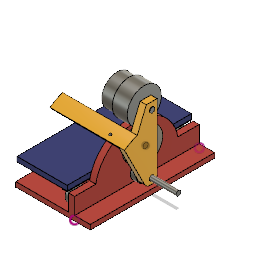
Second Design (Autodesk Fusion 360 design; units mm, degrees)
Autodesk Fusion 360 part; units mm, degrees
note: some values were not read from the file. Set by a fixed rule: which face or edge a step refers to.
sketch "Sketch1" plane through (0, 0, 0) normal (1, 0, 0) x (0, 0, -1)
  circle A0 centre (0, 0) radius 12.5
  line L0 (0, 0) -> (138.4704, 0)
  circle A1 centre (25, 0) radius 12.5
  circle A2 centre (65, 0) radius 27.5
  dimension "d1" = 25
  dimension "d2" = 25
  dimension "d3" = 55
  constraint coincident A0.centre L0.start
  constraint horizontal L0
  measures "d1" diameter of A0
  measures "d2" diameter of A1
  measures "d3" diameter of A2
extrude "Extrude1" add sketch "Sketch1" against normal blind 10 contours A0 | L0 A1 | L0 A1 makes body 1
sketch "Sketch2" plane through (0, 0, 0) normal (1, 0, 0) x (0, 0, -1)
  circle A0 centre (25, 0) radius 12.5
  line L0 (0, 0) -> (94.7994, 0)
  circle A1 centre (65, 0) radius 27.5
  dimension "d6" = 55
  constraint coincident L0.start origin
  constraint horizontal L0
  measures "d6" diameter of A1
extrude "Extrude2" add sketch "Sketch2" against normal blind 24 separate body contours L0 A1 | L0 A1 makes body 2
sketch "Sketch3" plane through (-24, 0, 0) normal (-1, 0, 0) x (0, 0, 1)
  circle A0 centre (-65, 0) radius 27.5
  circle A1 centre (-65, 0) radius 24.6188
  constraint concentric A0 A1
extrude "Extrude3" add sketch "Sketch3" along normal blind 20 contours A1 bodies 2
sketch "Sketch4" plane through (-10, 0, 0) normal (-1, 0, 0) x (0, 0, 1)
  circle A0 centre (0, 0) radius 12.5
  circle A1 centre (0, 0) radius 4
  dimension "d11" = 8
  constraint coincident A0.centre A1.centre
  measures "d11" diameter of A1
extrude "Extrude4" add sketch "Sketch4" along normal blind 50 separate body contours A1 makes body 3
sketch "Sketch5" plane through (0, 0, 0) normal (1, 0, 0) x (0, 0, -1)
  circle A0 centre (0, 0) radius 12.5
  circle A1 centre (0, 0) radius 4
  dimension "d14" = 8
  constraint coincident A0.centre A1.centre
  measures "d14" diameter of A1
extrude "Extrude5" add sketch "Sketch5" along normal blind 12 separate body contours A1 makes body 4
sketch "Sketch6" plane through (0, 0, 0) normal (1, 0, 0) x (0, 0, -1)
  circle A0 centre (25, 0) radius 12.5
  circle A1 centre (25, 0) radius 4
  dimension "d17" = 8
  constraint concentric A0 A1
  measures "d17" diameter of A1
extrude "Extrude6" add sketch "Sketch6" along normal blind 12 separate body contours A1 makes body 5
sketch "Sketch7" plane through (0, 0, 0) normal (1, 0, 0) x (0, 0, -1)
  circle A0 centre (65, 0) radius 27.5
  circle A1 centre (65, 0) radius 4
  dimension "d20" = 8
  constraint concentric A0 A1
  measures "d20" diameter of A1
extrude "Extrude7" add sketch "Sketch7" along normal blind 12 contours A1 bodies 2
sketch "Sketch8" plane through (12, 0, 0) normal (1, 0, 0) x (0, 0, -1)
  circle A0 centre (0, 0) radius 4
  line L0 (-9.1061, -8.5632) -> (91.0672, -8.5632)
  line L1 (91.0672, -8.5632) -> (91.0672, 8.7609)
  line L2 (91.0672, 8.7609) -> (-9.1061, 8.7609)
  line L3 (-9.1061, 8.7609) -> (-9.1061, -8.5632)
  circle A1 centre (0, 0) radius 12.5
  circle A2 centre (0, 0) radius 12.5
  circle A3 centre (65, 0) radius 27.5
  circle A4 centre (65, 0) radius 27.5
  constraint horizontal L0
  constraint vertical L1
  constraint horizontal L2
  constraint vertical L3
  constraint coincident L1.end A3
  constraint coincident L1.end A4
  constraint coincident L0.start A1
  constraint coincident L0.start A2
extrude "Extrude8" add sketch "Sketch8" against normal blind 10 contours L0 L2 L3 A1 A2 | L0 L2 A1 A2 A3 A4 | L0 L1 L2 A3 A4 bodies 2 4 5
sketch "Sketch9" plane through (12, 0, 0) normal (1, 0, 0) x (0, 0, -1)
  line L0 (91.0672, 8.7609) -> (-8.9161, 8.7609)
  arc A0 (-8.9161, 8.7609) -> (-9.1061, 8.5632) centre (0, 0) ccw
  line L1 (-9.1061, 8.5632) -> (-9.1061, -8.5632)
  line L2 (-9.1061, -8.5632) -> (91.0672, -8.5632)
  line L3 (91.0672, -8.5632) -> (91.0672, 8.7609)
  circle A1 centre (0, 0) radius 4
  dimension "d25" = 8
  constraint coincident A0.centre A1.centre
  measures "d25" diameter of A1
extrude "Extrude9" add sketch "Sketch9" along normal blind 1 contours A1 bodies 2
sketch "Sketch10" plane through (12, 0, 0) normal (1, 0, 0) x (0, 0, -1)
  circle A0 centre (0, 0) radius 4
  line L0 (91.0672, 8.7609) -> (-8.9161, 8.7609)
  arc A1 (-8.9161, 8.7609) -> (-9.1061, 8.5632) centre (0, 0) ccw
  line L1 (-9.1061, 8.5632) -> (-9.1061, -8.5632)
  line L2 (-9.1061, -8.5632) -> (91.0672, -8.5632)
  line L3 (91.0672, -8.5632) -> (91.0672, 8.7609)
  circle A2 centre (25, 0) radius 4
  circle A3 centre (25, 0) radius 4
  circle A4 centre (65, 0) radius 4
  circle A5 centre (65, 0) radius 4
  point P0 (21, 0)
  point P1 (61, 0)
  constraint tangent A2 A3
  constraint coincident A2 P0
  constraint tangent A4 A5
  constraint coincident A4 P1
extrude "Extrude10" add sketch "Sketch10" along normal blind 1 contours A2 A3 | A4 A5 bodies 2
move_face "OffsetFaces1" offset -23 1 faces at (-60, 0.0132, -1.2456) on bodies 3
move_face "OffsetFaces2" offset -26 1 faces at (-37, 0.7511, 1.1017) on bodies 3
move_face "OffsetFaces3" offset 1 1 faces at (-11, 0.7511, 1.1017) on bodies 3
sketch "Sketch11" plane through (-12, 0, 0) normal (-1, 0, 0) x (0, 0, 1)
  circle A0 centre (0, 0) radius 4
  circle A1 centre (0, 0) radius 35.5624
  constraint coincident A0.centre A1.centre
extrude "Extrude11" add sketch "Sketch11" along normal blind 10 separate body makes body 6
delete_face "DeleteFace1" 1 faces at (5.3333, 8.6516, 9.0222) on bodies 2
move_face "OffsetFaces4" offset 25 1 faces at (5.3333, 2.9862, 9.1061) on bodies 2
move_face "OffsetFaces5" offset 65 1 faces at (-12, 0.7511, 1.1017) on bodies 3
sketch "Sketch12" plane through (-22, 0, 0) normal (-1, 0, 0) x (0, 0, 1)
  circle A0 centre (0, 0) radius 4
  circle A1 centre (0, 0) radius 35.5624
  line L0 (-35.5624, 0) -> (35.5624, 0)
  line L1 (35.5624, 0) -> (35.5624, -45.6152)
  line L2 (35.5624, -45.6152) -> (-35.5624, -45.6152)
  line L3 (-35.5624, -45.6152) -> (-35.5624, 0)
  point P0 (-35.5624, 0)
  constraint perpendicular L0 L1
  constraint parallel L0 L2
  constraint parallel L1 L3
  constraint coincident A1 L0.end
  constraint coincident P0 L0.start
extrude "Extrude12" add sketch "Sketch12" against normal blind 10 contours A1 L1 L2 L3 bodies 6
copy_body "CopyPasteBodies1" bodies 1 makes body 7
move_body "Move1" bodies 7 to x (1, 0, 0) y (0, 1, 0) z (0, 0, 1) at (-35, 0, 0)
delete_face "DeleteFace2" 3 faces at (-38.3333, 10.5003, -18.2182) (-41.6667, -0.6231, -37.4845) (-45, 0.8046, -28.525) on bodies 7
sketch "Sketch13" plane through (12, 0, 0) normal (1, 0, 0) x (0, 0, -1)
  line L0 (-34.1061, 8.7609) -> (-34.1061, -8.5632)
  line L1 (-34.1061, -8.5632) -> (91.0672, -8.5632)
  line L2 (91.0672, -8.5632) -> (91.0672, 8.7609)
  line L3 (91.0672, 8.7609) -> (-34.1061, 8.7609)
  circle A0 centre (65, 0) radius 4
  circle A1 centre (25, 0) radius 4
  circle A2 centre (0, 0) radius 4
  line L4 (8.8225, 44.5071) -> (-8.8225, 44.5071)
  line L5 (-8.8225, 44.5071) -> (-8.8225, -44.5071)
  line L6 (-8.8225, -44.5071) -> (8.8225, -44.5071)
  line L7 (8.8225, -44.5071) -> (8.8225, 44.5071)
  line L8 (8.8225, 44.5071) -> (-8.8225, -44.5071) construction
  line L9 (-8.8225, 44.5071) -> (8.8225, -44.5071) construction
  constraint perpendicular L4 L5
  constraint parallel L4 L6
  constraint parallel L5 L7
  constraint horizontal L4
  constraint coincident L8 A2.centre
  constraint coincident L9 A2.centre
  constraint coincident A2.centre origin
extrude "Extrude13" add sketch "Sketch13" against normal blind 10 contours L3 L4 L5 L7 bodies 2
move_face "OffsetFaces6" offset -25 1 faces at (8.6667, 2.9862, 34.1061) on bodies 2
sketch "Sketch14" plane through (2, 0, 0) normal (-1, 0, 0) x (0, 0, 1)
  circle A0 centre (-25, 0) radius 4
  line L0 (9.1061, -8.5632) -> (9.1061, 8.7609)
  line L1 (9.1061, 8.7609) -> (8.8225, 8.7609)
  line L2 (8.8225, 8.7609) -> (8.8225, 44.5071)
  line L3 (8.8225, 44.5071) -> (-8.8225, 44.5071)
  line L4 (-8.8225, 44.5071) -> (-8.8225, 8.7609)
  line L5 (-8.8225, 8.7609) -> (-91.0672, 8.7609)
  line L6 (-91.0672, 8.7609) -> (-91.0672, -8.5632)
  line L7 (-91.0672, -8.5632) -> (9.1061, -8.5632)
  circle A1 centre (0, 0) radius 4
  circle A2 centre (-65, 0) radius 4
  line L8 (-8.8225, 44.5071) -> (8.8225, 44.5071)
  line L9 (8.8225, 44.5071) -> (8.8225, 36.5071)
  line L10 (8.8225, 36.5071) -> (-8.8225, 36.5071)
  line L11 (-8.8225, 36.5071) -> (-8.8225, 44.5071)
  dimension "d42" = 8
  constraint horizontal L8
  constraint vertical L9
  constraint horizontal L10
  constraint vertical L11
  constraint coincident L3.end L4.start
  measures "d42" distance of L3.end L10.end
extrude "Extrude14" add sketch "Sketch14" along normal blind 125 contours L2 L3 L4 L8 L9 L10 L11 bodies 2
move_body "Move2" bodies 1 2 to x (1, 0, 0) y (0, 0, 1) z (0, -1, 0) at (0, 0, 0)
delete_face "DeleteFace3" 3 faces at (-78, 2.9408, 44.5071) (-123, -2.9408, 39.1737) (8.6667, 8.8225, 29.925) on bodies 2
sketch "Sketch15" plane through (-22, 0, 0) normal (-1, 0, 0) x (0, 0, 1)
  circle A0 centre (0, 0) radius 4
  arc A1 (35.5624, 0) -> (-35.5624, 0) centre (0, 0) ccw
  line L0 (-35.5624, 0) -> (-35.5624, -45.6152)
  line L1 (-35.5624, -45.6152) -> (35.5624, -45.6152)
  line L2 (35.5624, -45.6152) -> (35.5624, 0)
  line L3 (0, 35.5624) -> (35.5624, 35.5624)
  line L4 (35.5624, 35.5624) -> (35.5624, -45.6152)
  line L5 (35.5624, -45.6152) -> (0, -45.6152)
  line L6 (0, -45.6152) -> (0, 35.5624)
  constraint horizontal L3
  constraint vertical L4
  constraint horizontal L5
  constraint vertical L6
  constraint coincident L1.end L2.start
  constraint midpoint A1 L3.start
extrude "Extrude15" add sketch "Sketch15" against normal blind 10 contours A1 L3 L4 bodies 6
sketch "Sketch16" plane through (-45, 0, 0) normal (-1, 0, 0) x (0, 0, 1)
  circle A0 centre (0, 0) radius 12.5
  line L0 (0, 12.5) -> (-100, 12.5)
  line L1 (-100, 12.5) -> (-100, 20.5)
  line L2 (-100, 20.5) -> (0, 20.5)
  line L3 (0, 20.5) -> (0, 12.5)
  point P0 (0, 12.5)
  dimension "d48" = 100
  dimension "d49" = 8
  constraint horizontal L0
  constraint vertical L1
  constraint horizontal L2
  constraint vertical L3
  constraint coincident P0 L0.start
  measures "d48" distance of P0 L0.end
  measures "d49" distance of P0 L2.end
extrude "Extrude16" add sketch "Sketch16" along normal blind 70 separate body contours L0 L1 L2 L3 makes body 8
move_face "OffsetFaces7" offset 100 1 faces at (-91.6667, 17.8333, 0) on bodies 8
move_body "Move3" bodies 8 to x (1, 0, 0) y (0, 1, 0) z (0, 0, 1) at (0, 1, 0)
move_body "Move4" bodies 8 to x (1, 0, 0) y (0, 1, 0) z (0, 0, 1) at (10, 0, 0)
move_face "OffsetFaces8" offset 11 1 faces at (-35, 16.1667, 33.3333) on bodies 8
move_face "OffsetFaces9" offset -15 1 faces at (5.3333, 91.0672, 2.9862) on bodies 2
move_face "OffsetFaces10" offset -25 1 faces at (-18.6667, -45.6152, 11.8541) on bodies 6
move_face "OffsetFaces11" offset 10 1 faces at (-15.3333, -1.8893, 35.5624) on bodies 6
sketch "Sketch17" plane through (-22, 0, 0) normal (-1, 0, 0) x (0, 0, 1)
  circle A0 centre (0, 0) radius 4
  arc A1 (0, 35.5624) -> (-35.5624, 0) centre (0, 0) ccw
  line L0 (-35.5624, 0) -> (-35.5624, -20.6152)
  line L1 (-35.5624, -20.6152) -> (45.5624, -20.6152)
  line L2 (45.5624, -20.6152) -> (45.5624, 35.5624)
  line L3 (45.5624, 35.5624) -> (0, 35.5624)
  line L4 (45.5624, 12.1225) -> (-35.5624, 12.1225)
  line L5 (-35.5624, 12.1225) -> (-35.5624, -20.6152)
  line L6 (-35.5624, -20.6152) -> (45.5624, -20.6152)
  line L7 (45.5624, -20.6152) -> (45.5624, 12.1225)
  constraint horizontal L4
  constraint vertical L5
  constraint horizontal L6
  constraint vertical L7
  constraint coincident L0.end L1.start
  constraint coincident L2 L4.start
extrude "Extrude17" add sketch "Sketch17" against normal blind 10 contours A1 L4 L5 bodies 6
move_face "OffsetFaces12" offset 20 1 faces at (-15.3333, -9.7026, -35.5624) on bodies 6
move_face "OffsetFaces13" offset 45 1 faces at (-15.3333, -9.7026, -55.5624) on bodies 6
sketch "Sketch18" plane through (0, 13.5, 0) normal (0, -1, 0) x (1, 0, 0)
  line L0 (-24, -100) -> (-24, 100)
  line L1 (-24, 100) -> (-105, 100)
  line L2 (-105, 100) -> (-105, -100)
  line L3 (-105, -100) -> (-24, -100)
  line L4 (-45, -12.5) -> (-35, -12.5)
  line L5 (-35, -12.5) -> (-35, 11.9)
  line L6 (-35, 11.9) -> (-45, 11.9)
  line L7 (-45, 11.9) -> (-45, -12.5)
  line L8 (-35, -12.5) -> (-35, 12.5)
  point P0 (-45, -12.5)
  constraint horizontal L4
  constraint vertical L5
  constraint horizontal L6
  constraint vertical L7
  constraint coincident L5.end L8
  constraint coincident P0 L4.start
extrude "Extrude18" add sketch "Sketch18" along normal blind 1 contours L4 L5 L6 L7 L8 bodies 8 7
move_face "OffsetFaces14" offset 100 1 faces at (-38.3333, 13.1667, 11.9) on bodies 8
move_face "OffsetFaces15" offset 100 1 faces at (-41.6667, 13.1667, -12.5) on bodies 8
move_body "Move5" bodies 2 to x (1, 0, 0) y (0, 1, 0) z (0, 0, 1) at (0, 30, 0)
delete_face "DeleteFace4" 2 faces at (-3.3333, 18.2182, 10.5003) (-6.6667, 37.4845, -0.6231) on bodies 1
delete_face "DeleteFace5" 4 faces at (12.3333, 33.995, 0.1994) (13, 29.8494, 0.6494) (12.3333, 58.995, 0.1994) (13, 53.7408, 0.1943) on bodies 2
sketch "Sketch19" plane through (2, 0, 0) normal (-1, 0, 0) x (0, 0, 1)
  circle A0 centre (0, 95) radius 4
  circle A1 centre (0, 30) radius 4
  circle A2 centre (0, 55) radius 4
  line L0 (-8.5632, 106.0672) -> (-8.5632, 20.8939)
  line L1 (-8.5632, 20.8939) -> (8.7609, 20.8939)
  line L2 (8.7609, 20.8939) -> (8.7609, 106.0672)
  line L3 (8.7609, 106.0672) -> (-8.5632, 106.0672)
  circle A3 centre (-0.0646, 39.9013) radius 27.5
  dimension "d65" = 55
  measures "d65" diameter of A3
extrude "Extrude19" add sketch "Sketch19" along normal blind 10 contours L0 L1 L2 A3 | L0 L1 L2 A3 bodies 1 2
sketch "Sketch20" plane through (0, 0, 0) normal (1, 0, 0) x (0, 0, -1)
  arc A0 (-1.2807, 12.4342) -> (1.321, 12.43) centre (0.0646, 39.9013) ccw
  arc A1 (-1.2807, 12.4342) -> (1.321, 12.43) centre (0, 0) ccw
  circle A2 centre (0, 0) radius 4
  dimension "d68" = 8
  constraint coincident A1.centre A2.centre
  measures "d68" diameter of A2
extrude "Extrude20" add sketch "Sketch20" along normal blind 55 contours A2 bodies 1
sketch "Sketch21" plane through (-12, 0, 0) normal (1, 0, 0) x (0, 0, -1)
  circle A0 centre (0, 0) radius 4
  line L0 (-45.5624, 35.5624) -> (-45.5624, -20.6152)
  line L1 (-45.5624, -20.6152) -> (100.5624, -20.6152)
  line L2 (100.5624, -20.6152) -> (100.5624, 12.1225)
  line L3 (100.5624, 12.1225) -> (33.4325, 12.1225)
  arc A1 (33.4325, 12.1225) -> (0, 35.5624) centre (0, 0) ccw
  line L4 (0, 35.5624) -> (-45.5624, 35.5624)
  circle A2 centre (0, 0) radius 67.0715
  constraint coincident A0.centre A1.centre
extrude "Extrude21" add sketch "Sketch21" against normal blind 10 contours L0 L1 L3 A1 L4 A2 picked at (-52.5148, 8.0924) bodies 6
sketch "Sketch22" plane through (-22, 0, 0) normal (-1, 0, 0) x (0, 0, 1)
  circle A0 centre (0, 0) radius 4
  arc A1 (-63.8248, -20.6152) -> (-65.9669, 12.1225) centre (0, 0) ccw
  line L0 (-65.9669, 12.1225) -> (-100.5624, 12.1225)
  line L1 (-100.5624, 12.1225) -> (-100.5624, -20.6152)
  line L2 (-100.5624, -20.6152) -> (-63.8248, -20.6152)
  circle A2 centre (0, 32.5) radius 11
  dimension "d73" = 22
  measures "d73" diameter of A2
extrude "Extrude22" add sketch "Sketch22" along normal blind 7 contours A2 bodies 6 8
delete_face "DeleteFace6" 4 faces at (-45, -1.3409, 2.8638) (-41.6667, 12.4858, -0.5948) (-41.6667, -0.6133, -12.4849) (-35, -1.3409, 2.8638) on bodies 6
delete_face "DeleteFace7" 1 faces at (-41.6667, 12.5, -37.5) on bodies 6
delete_face "DeleteFace8" 4 faces at (-41.6667, 13.1667, -112.5) (-45, 12.8333, 33.1333) (-41.6667, 13.5, -104.1667) (-38.3333, 12.5, -37.7) on bodies 6
sketch "Sketch23" plane through (-22, 0, 0) normal (-1, 0, 0) x (0, 0, 1)
  circle A0 centre (0, 32.5) radius 11
  circle A1 centre (0, 0) radius 4
  arc A2 (-63.8248, -20.6152) -> (-65.9669, 12.1225) centre (0, 0) ccw
  line L0 (-65.9669, 12.1225) -> (-100.5624, 12.1225)
  line L1 (-100.5624, 12.1225) -> (-100.5624, -20.6152)
  line L2 (-100.5624, -20.6152) -> (-63.8248, -20.6152)
  circle A3 centre (0, 0) radius 12.5
  dimension "d76" = 25
  constraint coincident A1.centre A2.centre
  measures "d76" diameter of A3
extrude "Extrude23" add sketch "Sketch23" along normal blind 10 contours A3 bodies 3 6
sketch "Sketch24" plane through (0, 13.5, 0) normal (0, -1, 0) x (1, 0, 0)
  line L0 (-105, -100) -> (-24, -100)
  line L1 (-24, -100) -> (-24, 100)
  line L2 (-24, 100) -> (-105, 100)
  line L3 (-105, 100) -> (-105, -100)
  line L4 (-24, -100) -> (-44.45, -100)
  line L5 (-44.45, -100) -> (-44.45, 100)
  line L6 (-44.45, 100) -> (-24, 100)
  line L7 (-24, 100) -> (-24, -100)
  constraint horizontal L4
  constraint vertical L5
  constraint horizontal L6
  constraint vertical L7
  constraint coincident L2 L5.end
  constraint coincident L0.end L1.start
extrude "Extrude24" add sketch "Sketch24" along normal blind 1 separate body contours L0 L1 L2 L4 L5 L6 L7 makes body 9
extrude "Extrude25" cut 1 faces at (-44.45, 13.1667, -33.3333) along direction (1, 0, 0) blind 13 on bodies 9 bodies 9
extrude "Extrude26" add 1 faces at (5.3333, 20.8939, 2.9862) along direction (0, -1, 0) blind 30 on bodies 1 bodies 1
sketch "Sketch25" plane through (2, 0, 0) normal (1, 0, 0) x (0, 0, -1)
  line L0 (8.5632, 66.0551) -> (8.5632, 13.7474)
  arc A0 (8.5632, 13.7474) -> (8.5632, 66.0551) centre (0.0646, 39.9013) ccw
  circle A1 centre (0.0646, 39.9013) radius 4
  dimension "d85" = 8
  constraint concentric A0 A1
  measures "d85" diameter of A1
sketch "Sketch26" plane through (12, 0, 0) normal (1, 0, 0) x (0, 0, -1)
  circle A0 centre (0, 0) radius 4
  circle A1 centre (0, 95) radius 4
  line L0 (-8.7609, 106.0672) -> (-8.7609, -9.1061)
  line L1 (-8.7609, -9.1061) -> (8.5632, -9.1061)
  line L2 (8.5632, -9.1061) -> (8.5632, 106.0672)
  line L3 (8.5632, 106.0672) -> (-8.7609, 106.0672)
  arc A2 (65.9669, 12.1225) -> (63.8248, -20.6152) centre (0, 0) ccw
  line L4 (0, 0) -> (-39.5306, 54.1841)
  line L5 (0, 95) -> (-39.5306, 54.1841)
  line L6 (0, 95) -> (0, 0)
  constraint coincident A0.centre A2.centre
  constraint coincident A2 L4.end
  constraint coincident A1.centre L5.start
extrude "Extrude27" add sketch "Sketch26" against normal blind 10 contours L0 A2 L4 | L0 A2 L5 bodies 1
sketch "Sketch27" plane through (12, 0, 0) normal (1, 0, 0) x (0, 0, -1)
  circle A0 centre (0, 0) radius 4
  circle A1 centre (0, 95) radius 4
  line L0 (-8.7609, 106.0672) -> (-8.7609, 85.9543)
  line L1 (-8.7609, 85.9543) -> (-39.5306, 54.1841)
  line L2 (-39.5306, 54.1841) -> (-8.7609, 12.0084)
  line L3 (-8.7609, 12.0084) -> (-8.7609, -9.1061)
  line L4 (-8.7609, -9.1061) -> (8.5632, -9.1061)
  line L5 (8.5632, -9.1061) -> (8.5632, 106.0672)
  line L6 (8.5632, 106.0672) -> (-8.7609, 106.0672)
  line L7 (-8.7609, 12.0084) -> (-64.8706, 88.9175)
  line L8 (-8.7609, 106.0672) -> (-47.8998, 65.6557)
  constraint coincident L2.end L3.start
  constraint parallel L2 L7
  constraint coincident L0.start L6.end
  constraint coincident L7 L8.end
  constraint parallel L1 L8
extrude "Extrude28" add sketch "Sketch27" against normal blind 10 contours L0 L1 L7 L8 bodies 1
sketch "Sketch28" plane through (12, 0, 0) normal (1, 0, 0) x (0, 0, -1)
  circle A0 centre (0, 0) radius 4
  circle A1 centre (0, 95) radius 4
  line L0 (-8.7609, 106.0672) -> (-47.8998, 65.6557)
  line L1 (-47.8998, 65.6557) -> (-8.7609, 12.0084)
  line L2 (-8.7609, 12.0084) -> (-8.7609, -9.1061)
  line L3 (-8.7609, -9.1061) -> (8.5632, -9.1061)
  line L4 (8.5632, -9.1061) -> (8.5632, 106.0672)
  line L5 (8.5632, 106.0672) -> (-8.7609, 106.0672)
  circle A2 centre (0, 0) radius 74.4025
  circle A3 centre (0, 0) radius 69
  line L6 (0, 0) -> (-28.3303, 85.8614)
  dimension "d90" = 138
  constraint concentric A0 A2
  constraint concentric A2 A3
  constraint coincident A0.centre A2.centre
  constraint midpoint L0 L6.end
  measures "d90" diameter of A3
extrude "Extrude29" add sketch "Sketch28" against normal blind 50 contours L1 A2 A3 L6 bodies 1
hole "Hole1" at (-17.2722, 64.4021, 37.2572) direction (0, -0.865591, -0.500752) diameter 4 depth 20 tip angle 118 bodies 1 3
sketch "Sketch29" plane through (2, 0, 0) normal (-1, 0, 0) x (0, 0, 1)
  circle A0 centre (0, 95) radius 4
  arc A1 (40.6672, 55.7421) -> (21.6203, 65.5253) centre (0, 0) ccw
  line L0 (21.6203, 65.5253) -> (23.3131, 70.6557)
  arc A2 (43.8513, 60.1066) -> (23.3131, 70.6557) centre (0, 0) ccw
  line L1 (43.8513, 60.1066) -> (47.8998, 65.6557)
  line L2 (47.8998, 65.6557) -> (8.7609, 106.0672)
  line L3 (8.7609, 106.0672) -> (-8.5632, 106.0672)
  line L4 (-8.5632, 106.0672) -> (-8.5632, 66.0551)
  arc A3 (27.3265, 37.4561) -> (-8.5632, 66.0551) centre (-0.0646, 39.9013) ccw
  line L5 (27.3265, 37.4561) -> (40.6672, 55.7421)
  line L6 (23.3131, 70.6557) -> (8.7609, 106.0672)
  constraint coincident L0.end A2.end
  constraint coincident L2.end L3.start
extrude "Extrude30" cut sketch "Sketch29" against normal blind 100 contours A2 L1 L2 L6 bodies 1
extrude "Extrude31" add 1 faces at (-38, 60.0592, 40.634) along direction (-1, 0, 0) blind 70 on bodies 1 bodies 1
sketch "Sketch30" plane through (-12, 0, 0) normal (1, 0, 0) x (0, 0, -1)
  circle A0 centre (0, 0) radius 4
  line L0 (63.8248, -20.6152) -> (100.5624, -20.6152)
  line L1 (100.5624, -20.6152) -> (100.5624, 12.1225)
  line L2 (100.5624, 12.1225) -> (65.9669, 12.1225)
  arc A1 (65.9669, 12.1225) -> (63.8248, -20.6152) centre (0, 0) ccw
  line L3 (100.5624, -20.6152) -> (-141.7236, -20.6152)
  constraint coincident L0.end L1.start
  constraint perpendicular L1 L3
extrude "Extrude32" cut sketch "Sketch30" against normal blind 40 contours A1 L3 bodies 3
extrude "Extrude33" add 1 faces at (-15.3333, -9.7026, -100.5624) along direction (0, 0, 1) up to surface (200.5624 mm away) on bodies 3 bodies 3
sketch "Sketch31" plane through (12, 0, 0) normal (1, 0, 0) x (0, 0, -1)
  arc A0 (-23.3131, 70.6557) -> (-43.8513, 60.1066) centre (0, 0) ccw
  line L0 (-43.8513, 60.1066) -> (-8.7609, 12.0084)
  line L1 (-8.7609, 12.0084) -> (-8.7609, -9.1061)
  line L2 (-8.7609, -9.1061) -> (8.5632, -9.1061)
  line L3 (8.5632, -9.1061) -> (8.5632, 106.0672)
  line L4 (8.5632, 106.0672) -> (-8.7609, 106.0672)
  line L5 (-8.7609, 106.0672) -> (-23.3131, 70.6557)
  circle A1 centre (0, 95) radius 4
  circle A2 centre (0, 0) radius 4
  line L6 (-43.8513, 60.1066) -> (-8.7609, -9.1061)
  constraint coincident A0.end L0.start
  constraint coincident L1.end L2.start
extrude "Extrude34" add sketch "Sketch31" against normal blind 10 contours L0 L1 L6 bodies 1
sketch "Sketch32" plane through (-22, 0, 0) normal (-1, 0, 0) x (0, 0, 1)
  circle A0 centre (0, 0) radius 12.5
  line L0 (-65.9669, 12.1225) -> (-100.5624, 12.1225)
  line L1 (-100.5624, 12.1225) -> (-100.5624, -20.6152)
  line L2 (-100.5624, -20.6152) -> (100, -20.6152)
  line L3 (100, -20.6152) -> (100, 12.1225)
  line L4 (100, 12.1225) -> (65.9669, 12.1225)
  arc A1 (65.9669, 12.1225) -> (-65.9669, 12.1225) centre (0, 0) ccw
  circle A2 centre (0, 32.5) radius 11
  circle A3 centre (-83.2647, -0.3775) radius 12.5
  dimension "d106" = 25
  measures "d106" diameter of A3
extrude "Extrude35" add sketch "Sketch32" along normal blind 10 separate body contours A3 makes body 10
sketch "Sketch33" plane through (-22, 0, 0) normal (-1, 0, 0) x (0, 0, 1)
  circle A0 centre (0, 0) radius 12.5
  line L0 (-65.9669, 12.1225) -> (-100.5624, 12.1225)
  line L1 (-100.5624, 12.1225) -> (-100.5624, -20.6152)
  line L2 (-100.5624, -20.6152) -> (100, -20.6152)
  line L3 (100, -20.6152) -> (100, 12.1225)
  line L4 (100, 12.1225) -> (65.9669, 12.1225)
  arc A1 (65.9669, 12.1225) -> (-65.9669, 12.1225) centre (0, 0) ccw
  circle A2 centre (0, 32.5) radius 11
  circle A3 centre (82.9835, -0.3775) radius 12.5
  dimension "d109" = 25
  measures "d109" diameter of A3
extrude "Extrude36" add sketch "Sketch33" along normal blind 10 separate body contours A3 makes body 11
sketch "Sketch34" plane through (-12, 0, 0) normal (1, 0, 0) x (0, 0, -1)
  circle A0 centre (0, 0) radius 4
  arc A1 (65.9669, 12.1225) -> (-65.9669, 12.1225) centre (0, 0) ccw
  line L0 (-65.9669, 12.1225) -> (-100, 12.1225)
  line L1 (-100, 12.1225) -> (-100, -20.6152)
  line L2 (100.5624, -20.6152) -> (100.5624, 12.1225)
  line L3 (100.5624, 12.1225) -> (65.9669, 12.1225)
extrude "Extrude37" add 1 faces at (-15.3333, -20.6152, -33.7083) along direction (0, -1, 0) blind 10 on bodies 3 bodies 3
sketch "Sketch35" plane through (-12, 0, 0) normal (1, 0, 0) x (0, 0, -1)
  circle A0 centre (0, 0) radius 4
  arc A1 (65.9669, 12.1225) -> (-65.9669, 12.1225) centre (0, 0) ccw
  line L0 (-65.9669, 12.1225) -> (-100, 12.1225)
  line L1 (-100, 12.1225) -> (-100, -30.6152)
  line L2 (-100, -30.6152) -> (100.5624, -30.6152)
  line L3 (100.5624, -30.6152) -> (100.5624, 12.1225)
  line L4 (100.5624, 12.1225) -> (65.9669, 12.1225)
  line L5 (-0.0202, -12.5) -> (100.5624, -12.5)
  line L6 (100.5624, -12.5) -> (100.5624, -22.5)
  line L7 (100.5624, -22.5) -> (-0.0202, -22.5)
  line L8 (-0.0202, -22.5) -> (-0.0202, -12.5)
  arc A2 (-1.2807, 12.4342) -> (1.321, 12.43) centre (0, 0) ccw
  line L9 (100.5624, -22.5) -> (-100, -22.5)
  line L10 (-100, -22.5) -> (-100, -14.5)
  line L11 (-100, -14.5) -> (100.5624, -14.5)
  line L12 (100.5624, -14.5) -> (100.5624, -22.5)
  dimension "d114" = 10
  dimension "d115" = 8
  constraint horizontal L5
  constraint vertical L6
  constraint horizontal L7
  constraint vertical L8
  constraint midpoint L5.start A2
  constraint horizontal L9
  constraint vertical L10
  constraint horizontal L11
  constraint vertical L12
  constraint coincident L1 L10.end
  measures "d114" distance of L5.start L7.end
  measures "d115" distance of L6.end L11.end
extrude "Extrude38" add sketch "Sketch35" along normal blind 25 separate body contours L1 L8 L9 L10 L11 | L3 L6 L7 L8 L9 L11 L12 makes body 12
extrude "Extrude39" add 1 faces at (13, -17.1667, -67.0349) along direction (-1, 0, 0) blind 120 on bodies 12 bodies 12 9 10 11 3
extrude "Extrude40" cut 1 faces at (-12, -25.205, 33.1459) along direction (-1, 0, 0) blind 35 on bodies 12 bodies 12
fillet "Fillet1" radius 10 1 edges at (7, -9.1061, 8.7609) on bodies 1
fillet "Fillet2" radius 8 1 edges at (7, -9.1061, -8.5632) on bodies 1
